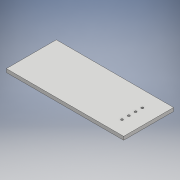
# Autodesk Inventor part: Zijplaat 4
Saved by Autodesk Inventor 2018.3 (Build 223284000, 284)
## iProperties
Created: 2020-11-10
Part Number: Zijplaat 4
Material: Generic
Document SubType Name: Modeling
Designer: daanv
Density: 1 g/cm^3
Appearance: Default
Author: daanv
Autodesk Inventor part; units mm, degrees
ref_plane "YZ Plane" through (0, 0, 0) normal (1, 0, 0) x (0, 1, 0)
ref_plane "XZ Plane" through (0, 0, 0) normal (0, 1, 0) x (-1, 0, 0)
ref_plane "XY Plane" through (0, 0, 0) normal (0, 0, 1) x (1, 0, 0)
sketch "Sketch1" plane through (0, 0, 0) normal (0, 0, 1) x (1, 0, 0)
  line L0 (0, 0) -> (0, 14.7)
  line L1 (0, 14.7) -> (34.5, 14.7)
  line L2 (34.5, 14.7) -> (34.5, 0)
  line L3 (34.5, 0) -> (0, 0)
  dimension "d0" = 14.7
  dimension "d1" = 34.5
  constraints: 8 end point, 3 perpendicular, 1 vertical
  measures "d0" distance of L0.start L0.end
  measures "d1" distance of L0.end L1.end
extrude "Extrusion1" add sketch "Sketch1" along normal blind 1
sketch "Sketch3" plane through (0, 0, 1) normal (0, 0, 1) x (1, 0, 0)
  point P0 (30, 10)
  point P1 (30, 8)
  point P2 (30, 6)
  point P3 (30, 4)
hole "Hole1" at (30, 10, 1) at (30, 8, 1) at (30, 6, 1) at (30, 4, 1) direction (0, 0, -1) diameter 0.65 end through all
body "Solid1"
